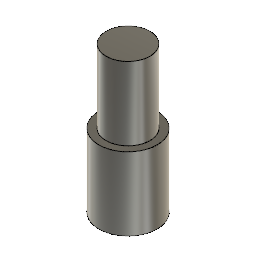
Pot Shaft Extender (Autodesk Fusion 360 design; units mm, degrees)
Autodesk Fusion 360 part; units mm, degrees
note: some values were not read from the file. Set by a fixed rule: which sketch regions a step uses.
sketch "Sketch1" plane through (0, 0, 0) normal (0, 0, 1) x (1, 0, 0)
  circle A0 centre (0, 0) radius 3
  circle A1 centre (0, 0) radius 4
  dimension "d1" = 6
  dimension "d4" = 8
  constraint coincident A0.centre A1.centre
  constraint concentric A0 A1
  measures "d1" diameter of A0
  measures "d4" diameter of A1
extrude "Extrude1" add sketch "Sketch1" along normal blind 12 contours A0 makes body 1
extrude "Extrude2" add sketch "Sketch1" against normal blind 8 separate body makes body 2
extrude "Extrude3" add sketch "Sketch1" along normal blind 2 bodies 1 2
named bodies: "extender 6"
